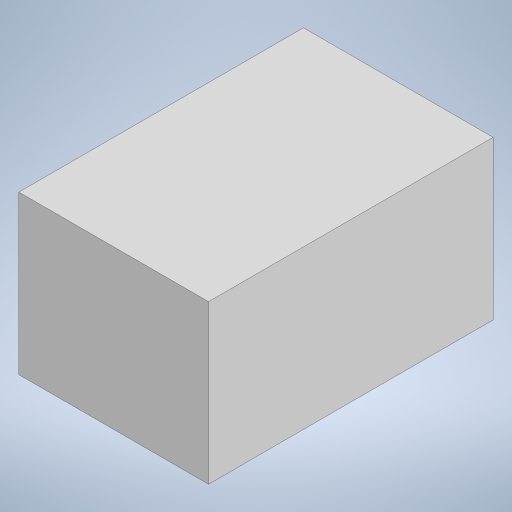
# Autodesk Inventor part: waist
Saved by Autodesk Inventor 2024.1 (Build 281209000, 209)
## iProperties
Created: 2024-10-10
Part Number: waist
Material: 一般
Document SubType Name: Modeling
Designer: hibik
Density: 1 g/cm^3
Appearance: 既定
Author: hibik
Autodesk Inventor part; units mm, degrees
ref_plane "YZ Plane" through (0, 0, 0) normal (1, 0, 0) x (0, 1, 0)
ref_plane "XZ Plane" through (0, 0, 0) normal (0, 1, 0) x (-1, 0, 0)
ref_plane "XY Plane" through (0, 0, 0) normal (0, 0, 1) x (1, 0, 0)
sketch "スケッチ1" plane through (0, 0, 0) normal (0, 1, 0) x (-1, 0, 0)
  line L0 (6, -9) -> (-6, -9)
  line L1 (-6, -9) -> (-6, 9)
  line L2 (-6, 9) -> (6, 9)
  line L3 (6, 9) -> (6, -9)
  line L4 (6, -9) -> (-6, 9) construction
  line L5 (-6, -9) -> (6, 9) construction
  point P0 (0, 0)
  dimension "d0" = 12
  dimension "d1" = 18
  constraints: 12 end point, 2 midpoint, 2 parallel, 1 horizontal, 1 perpendicular
  measures "d0" distance of L1.end L2.end
  measures "d1" distance of L0.end L1.end
extrude "押し出し1" add sketch "スケッチ1" along normal blind 10
